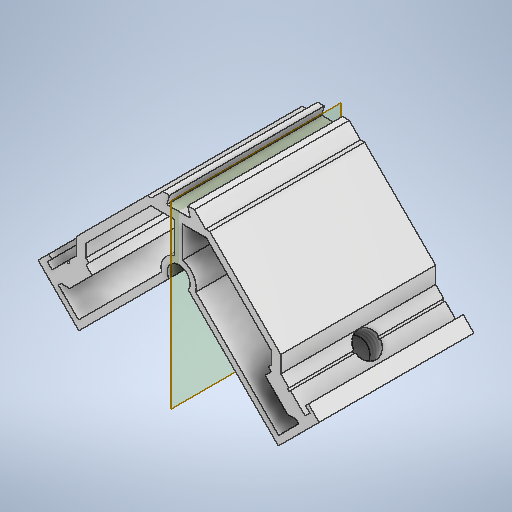
# Autodesk Inventor part: ESCUADRA
Saved by Autodesk Inventor 2025 (Build 290162000, 162)
## iProperties
Created: 2026-02-04
Part Number: ESCUADRA
Material: Aluminum
Document SubType Name: Modeling
Designer: Frank
Density: 2.7 g/cm^3
Appearance: Satin
Author: Frank
Autodesk Inventor part; units mm, degrees
ref_plane "YZ Plane" through (0, 0, 0) normal (1, 0, 0) x (0, 1, 0)
ref_plane "XZ Plane" through (0, 0, 0) normal (0, 1, 0) x (-1, 0, 0)
sketch "Sketch1" plane through (0, 0, 0) normal (0, 0, 1) x (1, 0, 0)
  line L0 (0, 0) -> (0, 7.4776)
  line L1 (0, 7.4776) -> (-5.7, 7.4776)
  line L2 (-5.7, 7.4776) -> (-21.2563, -8.0788)
  line L3 (-21.2563, -8.0788) -> (-21.2563, -11.0788)
  line L4 (-21.2563, -11.0788) -> (-20.5492, -11.7859)
  line L5 (-20.5492, -11.7859) -> (-21.2563, -12.493)
  line L6 (-21.2563, -12.493) -> (-19.7664, -13.983)
  line L7 (-19.7664, -13.983) -> (-25.1404, -19.357)
  line L8 (-25.1404, -19.357) -> (-27.1017, -19.2987)
  line L9 (-27.1017, -19.2987) -> (-27.8088, -20.0059)
  line L10 (-27.8088, -20.0059) -> (-23.0005, -24.8142)
  line L11 (-23.0005, -24.8142) -> (-3.2015, -5.0152)
  line L12 (-1.88, 9.6426) -> (-1.2574, 11.8658)
  line L13 (-1.2574, 11.8658) -> (-2.8574, 11.8658)
  line L14 (-2.8574, 11.8658) -> (-5.5444, 9.1788)
  line L15 (-23.5149, -7.7918) -> (-6.5444, 9.1788)
  line L16 (-6.5444, 9.1788) -> (-5.5444, 9.1788)
  line L17 (-23.5149, -7.7918) -> (-23.5149, -11.7918)
  line L18 (-29.3132, -17.5901) -> (-23.5149, -11.7918)
  line L19 (-29.3132, -17.5901) -> (-30.4446, -16.4587)
  line L20 (-30.4446, -16.4587) -> (-29.4153, -15.4295)
  line L21 (-29.4153, -15.4295) -> (-30.1224, -14.7223)
  line L22 (-30.1224, -14.7223) -> (-32.668, -17.2679)
  line L23 (-32.668, -17.2679) -> (-22.9298, -27.0062)
  line L24 (-22.9298, -27.0062) -> (-1.4337, -5.5102)
  line L25 (0.92, 16.812) -> (0.92, -19.9546) construction
  line L26 (1.84, 0) -> (1.84, 7.4776)
  line L27 (1.84, 7.4776) -> (7.54, 7.4776)
  line L28 (7.54, 7.4776) -> (23.0963, -8.0788)
  line L29 (23.0963, -8.0788) -> (23.0963, -11.0788)
  line L30 (23.0963, -11.0788) -> (22.3892, -11.7859)
  line L31 (22.3892, -11.7859) -> (23.0963, -12.493)
  line L32 (23.0963, -12.493) -> (21.6064, -13.983)
  line L33 (21.6064, -13.983) -> (26.9804, -19.357)
  line L34 (26.9804, -19.357) -> (28.9417, -19.2987)
  line L35 (28.9417, -19.2987) -> (29.6488, -20.0059)
  line L36 (29.6488, -20.0059) -> (24.8405, -24.8142)
  line L37 (24.8405, -24.8142) -> (5.0415, -5.0152)
  line L38 (3.72, 9.6426) -> (3.0974, 11.8658)
  line L39 (3.0974, 11.8658) -> (4.6974, 11.8658)
  line L40 (4.6974, 11.8658) -> (7.3844, 9.1788)
  line L41 (25.3549, -7.7918) -> (8.3844, 9.1788)
  line L42 (8.3844, 9.1788) -> (7.3844, 9.1788)
  line L43 (25.3549, -7.7918) -> (25.3549, -11.7918)
  line L44 (31.1532, -17.5901) -> (25.3549, -11.7918)
  line L45 (31.1532, -17.5901) -> (32.2846, -16.4587)
  line L46 (32.2846, -16.4587) -> (31.2553, -15.4295)
  line L47 (31.2553, -15.4295) -> (31.9624, -14.7223)
  line L48 (31.9624, -14.7223) -> (34.508, -17.2679)
  line L49 (34.508, -17.2679) -> (24.7698, -27.0062)
  line L50 (24.7698, -27.0062) -> (3.2737, -5.5102)
  line L51 (-1.88, 9.6426) -> (3.72, 9.6426)
  arc A0 (3.2737, -5.5102) -> (-1.4337, -5.5102) centre (0.92, -4.1167) ccw
  arc A1 (5.0415, -5.0152) -> (1.84, 0) centre (0.92, -4.1167) ccw
  arc A2 (0, 0) -> (-3.2015, -5.0152) centre (0.92, -4.1167) ccw
  point P0 (-22.4534, -16.67)
  dimension "d1" = 5.7
  dimension "d2" = 135
  dimension "d3" = 22
  dimension "d13" = 3
  dimension "d14" = 28
  dimension "d22" = 1.6
  dimension "d23" = 3.8
  dimension "d24" = 1
  dimension "d25" = 24
  dimension "d30" = 4
  dimension "d34" = 3.6
  dimension "d36" = 1.5
  dimension "d38" = 1.6
  dimension "d47" = 1.84
  dimension "d55" = 8.2
  dimension "d56" = 1.6
  dimension "d57" = 1
  dimension "d59" = 7.6
  dimension "d61" = 1
  dimension "d62" = 6.8
  dimension "d72" = 30.4
  dimension "d74" = 13.772
  dimension "d75" = 4.2
  dimension "d76" = 5.6
  dimension "d77" = 1.8
  dimension "d78" = 1
  dimension "d80" = 90
  dimension "d89" = 7.4776
  constraints: 104 end point, 27 symmetric about line, 10 perpendicular, 7 point on circle, 6 parallel, 3 centre point, 3 point on line, 3 vertical, 2 horizontal, 1 midpoint
  measures "d1" distance of L0.end L1.end
  measures "d2" angle of L1 L2
  measures "d3" distance of L1.end L2.end
  measures "d13" distance of L2.end L3.end
  measures "d14" distance of L11.end L10.end
  measures "d22" distance of L12.end L13.end
  measures "d23" distance of L13.end L14.end
  measures "d24" distance of L15.end L14.end
  measures "d25" distance of L15.start L15.end
  measures "d30" distance of L15.start L17.end
  measures "d34" distance of L21.end L22.end
  measures "d36" distance between parallel lines of L10 L23
  measures "d38" distance between parallel lines of L11 L24
  measures "d47" distance between parallel lines of L26 L0
  measures "d55" distance of L18.start L17.end
  measures "d56" distance of L18.start L19.end
  measures "d57" distance of L20.end L21.end
  measures "d59" distance of L6.end L7.end
  measures "d61" distance of L8.end L9.end
  measures "d62" distance of L9.end L10.end
  measures "d72" distance of L24.end L23.end
  measures "d74" distance of L22.end L23.end
  measures "d75" distance from line of L18 point (-22.453, -16.67)
  measures "d76" distance of L12.start L38.start
  measures "d77" distance between parallel lines of L15 L2
  measures "d78" distance of L3.end L4.end
  measures "d80" angle of L50 L24
  measures "d89" distance of L26.start L26.end
extrude "Extrusion1" add sketch "Sketch1" against normal blind 37
ref_plane "Work Plane2" through (31.1532, -17.5901, -37) normal (0.7071, 0.7071, 0) x (-0.7071, 0.7071, 0)
sketch "Sketch3" plane through (31.1532, -17.5901, -37) normal (0.7071, 0.7071, 0) x (-0.7071, 0.7071, 0)
  circle A0 centre (5.2, 18.5) radius 3
  line L0 (0, 37) -> (8.2, 37) projected
  line L1 (8.2, 37) -> (8.2, 0) projected
  point P0 (34.4667, 37)
  dimension "d65" = 18.5
  dimension "d67" = 6
  constraints: 1 centre point, 1 tangent
  measures "d65" distance from line of L0 A0.centre
  measures "d67" diameter of A0
extrude "Extrusion2" cut sketch "Sketch3" against normal blind 6
thread "Thread1" size "M6x1" class "6H" standard "ANSI Metric M Profile" full length
ref_plane "Work Plane4" through (0.92, 19.6401, -37) normal (-1, 0, 0) x (0, 0, -1)
mirror "Mirror2" about plane through (0.92, 19.6401, -37) normal (-1, 0, 0) of "Extrusion2"
thread "Thread2" size "M6x1" class "6H" standard "ANSI Metric M Profile" full length
sketch "Sketch4" plane through (31.1532, -17.5901, -37) normal (0.7071, 0.7071, 0) x (-0.7071, 0.7071, 0)
  line L0 (4.95, 0) -> (4.95, 37)
  line L1 (27.3556, 0) -> (-0.6444, 0) projected
  line L2 (0, 37) -> (8.2, 37) projected
  line L3 (5.45, 0) -> (5.45, 37)
  line L4 (8.2, 37) -> (8.2, 18.5) projected
  line L5 (5.45, 37) -> (4.95, 37)
  line L6 (5.45, 0) -> (4.95, 0)
  point P0 (34.4667, 37)
  point P1 (4.95, 0)
  dimension "d84" = 2.75
  dimension "d85" = 0.5
  constraints: 8 end point, 3 point on line, 2 horizontal, 1 perpendicular, 1 vertical
  measures "d84" distance between parallel lines of L4 L3
  measures "d85" distance between parallel lines of L3 L0
extrude "Extrusion3" cut sketch "Sketch4" against normal blind 0.5
mirror "Mirror3" about plane through (0.92, 19.6401, -37) normal (-1, 0, 0) of "Extrusion3"
body "Solid1"
